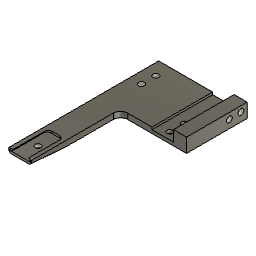
rail_NHP to 2mm rail adapter - long reach v34 (Autodesk Fusion 360 design; units mm, degrees)
Autodesk Fusion 360 part; units mm, degrees
note: some values were not read from the file. Set by a fixed rule: which sketch regions a step uses.
sketch "Sketch1" plane through (0, 0, 0) normal (0, 1, 0) x (1, 0, 0)
  line L0 (-12.4, 0.775) -> (12.4, 0.775)
  line L1 (12.4, 0.775) -> (12.4, -0.775)
  line L2 (12.4, -0.775) -> (-12.4, -0.775)
  line L3 (-12.4, -0.775) -> (-12.4, 0.775)
  line L4 (-12.4, 0.775) -> (12.4, -0.775) construction
  line L5 (12.4, 0.775) -> (-12.4, -0.775) construction
  dimension "d1" = 24.8
  dimension "d2" = 1.55
  constraint horizontal L0
  constraint perpendicular L0 L1
  constraint parallel L0 L2
  constraint parallel L1 L3
  constraint coincident L4 origin
  constraint coincident L5 origin
  measures "d1" distance of L1.end L2.end
  measures "d2" distance of L0.end L1.end
extrude "Extrude1" add sketch "Sketch1" along normal mid plane 17
sketch "Sketch4" plane through (0, 8.5, 0) normal (0, 1, 0) x (-1, 0, 0)
  line L0 (12.4, -0.775) -> (12.4, 0.775)
  line L1 (12.4, 0.775) -> (-12.4, 0.775)
  line L2 (-12.4, 0.775) -> (-12.4, -0.775)
  line L3 (-12.4, -0.775) -> (12.4, -0.775)
  line L4 (7.0918, 0.775) -> (6.7692, 0.2162)
  line L5 (6.7692, 0.2162) -> (11.6308, 0.2162)
  line L6 (11.6308, 0.2162) -> (11.3082, 0.775)
  point P0 (9.2, 0.2162)
  dimension "d11" = 60
  dimension "d12" = 60
  dimension "d13" = 4.2164
  dimension "d14" = 0.5588
  dimension "d47" = 3.2
  constraint coincident L1 L4.start
  constraint parallel L1 L5
  constraint coincident L1 L6.end
  constraint midpoint L5 P0
  measures "d11" angle of L4 L5
  measures "d12" angle of L5 L6
  measures "d13" distance of L4.start L6.end
  measures "d14" distance of L4.start L5
  measures "d47" distance of L0 P0
extrude "Extrude3" cut sketch "Sketch4" against normal up to surface (17 mm away) contours L1 L4 L5 L6
sketch "Sketch2" plane through (0, 8.5, 0) normal (0, 1, 0) x (-1, 0, 0)
  line L0 (7.0918, 0.775) -> (-12.4, 0.775)
  line L1 (-12.4, 0.775) -> (-12.4, -0.775)
  line L2 (-12.4, -0.775) -> (12.4, -0.775)
  line L3 (12.4, -0.775) -> (12.4, 0.775)
  line L4 (-2.7118, 0.141) -> (-8.7318, 0.141)
  line L5 (-8.7318, 0.141) -> (-8.7318, 0.775)
  line L6 (-8.7318, 0.775) -> (-2.7118, 0.775)
  line L7 (-2.7118, 0.775) -> (-2.7118, 0.141)
  line L8 (6.7692, 0.2162) -> (7.0918, 0.775)
  line L9 (12.4, 0.775) -> (11.3082, 0.775)
  line L10 (11.3082, 0.775) -> (11.6308, 0.2162)
  line L11 (11.6308, 0.2162) -> (6.7692, 0.2162)
  dimension "d5" = 6.02
  dimension "d6" = 0.634
  dimension "d50" = 9.481
  constraint horizontal L4
  constraint vertical L5
  constraint horizontal L6
  constraint vertical L7
  constraint collinear L0 L6
  measures "d5" distance of L5.end L6.end
  measures "d6" distance of L4.end L5.end
  measures "d50" distance of L7 L8.start
extrude "Extrude2" cut sketch "Sketch2" against normal up to surface (17 mm away) contours L0 L4 L5 L6 L7
sketch "Sketch6" plane through (0, 0, -0.775) normal (0, 0, -1) x (-1, 0, 0)
  line L0 (5.6836, 7) -> (5.6836, -7)
  line L1 (5.6836, -7) -> (6.75, -7)
  line L2 (6.75, -7) -> (6.75, 7)
  line L3 (6.75, 7) -> (5.6836, 7)
  line L4 (-0.15, 7) -> (-6.25, 7)
  line L5 (-5.7218, -6.5) -> (-5.7218, -2.5)
  line L6 (12.4, -8.5) -> (12.4, 8.5)
  line L7 (12.4, 8.5) -> (-12.4, 8.5)
  line L8 (-12.4, 8.5) -> (-12.4, -8.5)
  line L9 (-12.4, -8.5) -> (12.4, -8.5)
  line L10 (-8.7318, -8.5, -0.916) -> (-2.7118, -8.5, -0.916)
  line L11 (-2.7118, -8.5) -> (-8.7318, -8.5)
  line L12 (-8.7318, -8.5) -> (-8.7318, 8.5)
  line L13 (-8.7318, 8.5) -> (-2.7118, 8.5)
  line L14 (-2.7118, 8.5) -> (-2.7118, -8.5)
  point P0 (-5.7218, 7)
  point P1 (-5.7218, -2.5)
  point P2 (-5.7218, -6.5)
  point P3 (6.75, 0)
  point P4 (-5.7218, -4.5)
  point P5 (-5.7218, -8.5)
  point P6 (-5.7218, -8.5)
  dimension "d22" = 4
  dimension "d51" = 2
  constraint vertical P1 P2
  constraint midpoint L2 P3
  constraint coincident P2 L5.start
  constraint coincident P1 L5.end
  constraint midpoint L5 P4
  constraint vertical P0 P1
  constraint midpoint L11 P6
  constraint vertical P4 P6
  measures "d22" distance of P1 P2
  measures "d51" distance of P2 L9
hole "Hole2" at (5.7218, -2.5, -0.775) at (5.7218, -6.5, -0.775) direction (0, 0, 1) diameter 1.6 depth 3.517 tip angle 118
sketch "Sketch7" plane through (0, 0, -0.775) normal (0, 0, -1) x (-1, 0, 0)
  line L0 (5.6836, 7) -> (5.6836, -7)
  line L1 (5.6836, -7) -> (6.75, -7)
  line L2 (6.75, -7) -> (6.75, 7)
  line L3 (6.75, 7) -> (5.6836, 7)
  line L4 (-6.25, -7) -> (-0.15, -7)
  circle A0 centre (-5.7218, -2.5) radius 0.8
  circle A1 centre (-5.7218, -6.5) radius 0.8
  line L5 (12.4, -8.5) -> (12.4, 8.5)
  line L6 (12.4, 8.5) -> (-12.4, 8.5)
  line L7 (-12.4, 8.5) -> (-12.4, -8.5)
  line L8 (-12.4, -8.5) -> (12.4, -8.5)
  point P0 (-3.2, -7)
  point P1 (-3.2, -4.5)
  dimension "d26" = 2.5
  constraint midpoint L4 P0
  constraint vertical P0 P1
  measures "d26" distance of P0 P1
hole "Hole3" [suppressed]
thread "Thread3" [suppressed]
extrude "Extrude4" add 1 faces at (11.1773, -2.8333, 0.775) along direction (0, 0, 1) blind 2.4
sketch "Sketch10" plane through (12.4, 0, 0) normal (1, 0, 0) x (0, 1, 0)
  line L0 (-8.5, -0.775) -> (8.5, -0.775)
  line L1 (8.5, -0.775) -> (8.5, 3.175)
  line L2 (8.5, 3.175) -> (-8.5, 3.175)
  line L3 (-8.5, 3.175) -> (-8.5, -0.775)
  point P0 (3.5, 1.475)
  dimension "d54" = 2.25
  dimension "d59" = 12
  measures "d54" distance of L0 P0
  measures "d59" distance of L3 P0
hole "Hole6" at (12.4, 3.5, 1.475) direction (-1, 0, 0) diameter 1.623 depth 6.5 tip angle 118
thread "Thread6" "ISO Metric profile 2.0 M2x0.4 6H"
sketch "Sketch11" plane through (0, 8.5, 0) normal (0, 1, 0) x (-1, 0, 0)
  line L0 (11.6308, 0.2162) -> (6.7692, 0.2162)
  line L1 (7.0918, 0.775) -> (-2.7118, 0.775)
  line L2 (-2.7118, 0.775) -> (-2.7118, 0.141)
  line L3 (-2.7118, 0.141) -> (-8.7318, 0.141)
  line L4 (-8.7318, 0.141) -> (-8.7318, 3.175)
  line L5 (-8.7318, 3.175) -> (-12.4, 3.175)
  line L6 (-12.4, 3.175) -> (-12.4, -0.775)
  line L7 (-12.4, -0.775) -> (12.4, -0.775)
  line L8 (12.4, -0.775) -> (12.4, 0.775)
  line L9 (12.4, 0.775) -> (11.3082, 0.775)
  line L10 (11.3082, 0.775) -> (11.6308, 0.2162)
  line L11 (6.7692, 0.2162) -> (7.0918, 0.775)
  point P0 (-9.7318, 1.675)
  dimension "d60" = 1.5
  dimension "d61" = 1
  measures "d60" distance of L5 P0
  measures "d61" distance of L4 P0
hole "Hole7" at (9.7318, 8.5, 1.675) direction (0, -1, 0) diameter 0.8 depth 3 tip angle 118
sketch "Sketch12" plane through (12.4, 0, 0) normal (1, 0, 0) x (0, 1, 0)
  circle A0 centre (3.5, 1.475) radius 0.8115
  line L0 (-8.5, -0.775) -> (8.5, -0.775)
  line L1 (8.5, -0.775) -> (8.5, 3.175)
  line L2 (8.5, 3.175) -> (-8.5, 3.175)
  line L3 (-8.5, 3.175) -> (-8.5, -0.775)
  line L4 (8.5, 2.075) -> (8.5, 1.275)
  line L5 (5.5, 2.075) -> (5.5, 1.275)
  point P0 (6.75, 1.675)
  point P1 (8.5, 1.675)
  dimension "d66" = 1.75
  constraint midpoint L4 P1
  constraint horizontal P0 P1
  measures "d66" distance of P0 P1
hole "Hole8" at (12.4, 6.75, 1.675) direction (-1, 0, 0) diameter 1.623 depth 2.6 tip angle 118
thread "Thread7" "ISO Metric profile 2.0 M2x0.4 6H"
fillet "Fillet1" [suppressed]
sketch "Sketch13" plane through (0, -8.5, 0) normal (0, -1, 0) x (1, 0, 0)
  line L0 (8.7318, 3.175) -> (8.7318, 0.141)
  line L1 (8.7318, 0.141) -> (2.7118, 0.141)
  line L2 (2.7118, 0.141) -> (2.7118, 0.775)
  line L3 (2.7118, 0.775) -> (-7.0918, 0.775)
  line L4 (-7.0918, 0.775) -> (-6.7692, 0.2162)
  line L5 (-6.7692, 0.2162) -> (-11.6308, 0.2162)
  line L6 (-11.6308, 0.2162) -> (-11.3082, 0.775)
  line L7 (-11.3082, 0.775) -> (-12.4, 0.775)
  line L8 (-12.4, 0.775) -> (-12.4, -0.775)
  line L9 (-12.4, -0.775) -> (12.4, -0.775)
  line L10 (12.4, -0.775) -> (12.4, 3.175)
  line L11 (12.4, 3.175) -> (8.7318, 3.175)
  line L12 (2.7118, 0.141) -> (2.7118, -0.775)
  line L13 (-6.0918, 0.775) -> (-6.0918, -0.775)
  dimension "d78" = 1
  constraint coincident L1.end L2.start
  constraint coincident L9 L12.end
  constraint perpendicular L9 L12
  constraint coincident L3 L13.start
  constraint coincident L9 L13.end
  constraint perpendicular L9 L13
  measures "d78" distance of L3.end L13
extrude "Extrude5" add sketch "Sketch13" along normal blind 25 contours L3 L4 L5 L6 L7 L8 L9 L13
sketch "Sketch5" plane through (0, 0, -0.775) normal (0, 0, -1) x (1, 0, 0)
  line L0 (-12.4, -8.5) -> (12.4, -8.5)
  line L1 (12.4, -8.5) -> (12.4, 8.5)
  line L2 (12.4, 8.5) -> (-6.0918, 8.5)
  line L3 (-12.4, 33.5) -> (-12.4, -8.5)
  circle A0 centre (5.7218, 2.5) radius 0.8
  circle A1 centre (5.7218, 6.5) radius 0.8
  line L4 (-6.0918, 33.5) -> (-12.4, 33.5)
  line L5 (-6.7692, 33.5) -> (-11.6308, 33.5)
  line L6 (-6.0918, 8.5) -> (-6.0918, 33.5)
  point P0 (-9.2, 33.5)
  point P1 (-9.2, 28.5)
  dimension "d72" = 5
  constraint vertical P0 P1
  constraint midpoint P0 L5
  measures "d72" distance of P1 L4
hole "Hole1" at (-9.2, -28.5, -0.775) direction (0, 0, 1) diameter 1.623 end through all
thread "Thread1" "ISO Metric profile 2.0 M2x0.4 6H"
sketch "Sketch14" plane through (-6.0918, 0, 0) normal (1, 0, 0) x (0, 1, 0)
  line L0 (-8.5, 0.243) -> (8.5, 0.243)
  line L1 (8.5, 0.243) -> (8.5, 0.875)
  line L2 (8.5, 0.875) -> (-8.5, 0.875)
  line L3 (-8.5, 0.875) -> (-8.5, 0.243)
  line L4 (-33.5, -0.425) -> (-29.5, -0.775)
  line L5 (-8.5, -0.775) -> (-8.5, 0.775)
  line L6 (-8.5, 0.775) -> (-33.5, 0.775)
  line L7 (-33.5, 0.775) -> (-33.5, -0.775)
  line L8 (-33.5, -0.775) -> (-8.5, -0.775)
  dimension "d88" = 4
  dimension "d89" = 0.35
  constraint coincident L4.end L8
  constraint coincident L4.start L7
  measures "d88" distance of L4.end L7.end
  measures "d89" distance of L4.start L7.end
extrude "Extrude6" cut sketch "Sketch14" against normal through all contours L4 L7 L8
fillet "Fillet2" radius 0.5 2 edges at (-11.4695, -33.5, 0.4956) (-6.9305, -33.5, 0.4956)
sketch "Sketch15" plane through (0, 8.5, 0) normal (0, 1, 0) x (-1, 0, 0)
  circle A0 centre (-9.7318, 1.675) radius 0.4
  line L0 (-8.7318, 0.141) -> (-8.7318, 3.175)
  line L1 (-8.7318, 3.175) -> (-12.4, 3.175)
  line L2 (-12.4, 3.175) -> (-12.4, -0.775)
  line L3 (-12.4, -0.775) -> (12.4, -0.775)
  line L4 (12.4, -0.775) -> (12.4, 0.775)
  line L5 (12.4, 0.775) -> (11.3082, 0.775)
  line L6 (11.3082, 0.775) -> (11.6308, 0.2162)
  line L7 (11.6308, 0.2162) -> (6.7692, 0.2162)
  line L8 (6.7692, 0.2162) -> (7.0918, 0.775)
  line L9 (7.0918, 0.775) -> (-2.7118, 0.775)
  line L10 (-2.7118, 0.775) -> (-2.7118, 0.141)
  line L11 (-2.7118, 0.141) -> (-8.7318, 0.141)
  line L12 (7.0918, 0.775) -> (11.3082, 0.775)
  constraint coincident L8.end L9.start
  constraint coincident L5.end L6.start
extrude "Extrude7" add sketch "Sketch15" against normal blind 32 contours L6 L7 L8 L12
sketch "Sketch16" plane through (0, 0, 0.775) normal (0, 0, 1) x (-1, 0, 0)
  ellipse E0 centre (11.8856, 33) end of major axis (11.3082, 33) minor radius 0.5 (11.8856, 33.5) -> (11.3082, 33) ccw
  line L0 (11.3082, 33) -> (11.3082, 23.5)
  line L1 (11.3082, 23.5) -> (7.0918, 23.5)
  line L2 (7.0918, 23.5) -> (7.0918, 33)
  ellipse E1 centre (6.5144, 33) end of major axis (7.0918, 33) minor radius 0.5 (7.0918, 33) -> (6.5144, 33.5) ccw
  line L3 (6.5144, 33.5) -> (6.0918, 33.5)
  line L4 (6.0918, 33.5) -> (6.0918, 8.5)
  line L5 (6.0918, 8.5) -> (-2.7118, 8.5)
  line L6 (-2.7118, 8.5) -> (-2.7118, -8.5)
  line L7 (-2.7118, -8.5) -> (12.4, -8.5)
  line L8 (12.4, -8.5) -> (12.4, 33.5)
  line L9 (12.4, 33.5) -> (11.8856, 33.5)
  point P0 (9.2, 23.5)
  point P1 (9.2, -4.5)
  point P2 (9.2, -0.5)
  dimension "d81" = 4
  dimension "d85" = 4
  constraint midpoint L1 P0
  constraint vertical P0 P1
  constraint vertical P1 P2
  measures "d81" distance of L7 P1
  measures "d85" distance of P1 P2
hole "Hole9" at (-9.2, 4.5, 0.775) at (-9.2, 0.5, 0.775) direction (0, 0, -1) diameter 1.623 depth 9 tip angle 118
thread "Thread8" "ISO Metric profile 2.0 M2x0.4 6H"
fillet "Fillet3" radius 1 2 edges at (-6.9305, -23.5, 0.4956) (-11.4695, -23.5, 0.4956)
fillet "Fillet4" radius 2 1 edges at (-6.0918, -8.5, 0)
chamfer "Chamfer1" distance 0.5 angle 45 3 edges at (-6.0918, -31.5, -0.6) (-12.4, -31.5, -0.6) (-12.4, -10.5, -0.775)
equation "d6 = 0.75 mm - 0.116 mm"
